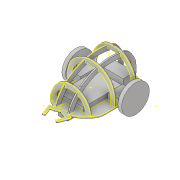
# Autodesk Inventor part: Chasis
Saved by Autodesk Inventor 2019 (Build 230136000, 136)
## iProperties
Created: 2019-02-16
Part Number: Chasis
Material: Generic
Document SubType Name: Modeling
Designer: carlg
Density: 1 g/cm^3
Appearance: Default
Author: carlg
Autodesk Inventor part; units mm, degrees
sketch "Sketch1" plane through (0, 0, 0) normal (0, 1, 0) x (-1, 0, 0)
  line L0 (0, 0) -> (-55.3, 0)
  line L1 (-55.3, 0) -> (-55.3, -83.15)
  line L2 (-55.3, -83.15) -> (0, -83.15)
  line L3 (0, -83.15) -> (0, 0)
  line L4 (-27.65, -83.15) -> (-27.65, 0) construction
  line L5 (-55.3, -83.15) -> (-55.3, 0)
  line L6 (-52.05, -89.15) -> (-3.25, -89.15)
  line L7 (-3.25, -89.15) -> (-3.25, -115.15)
  line L8 (-3.25, -115.15) -> (-52.05, -115.15)
  line L9 (-52.05, -115.15) -> (-52.05, -89.15)
  line L10 (-17.49, 2) -> (-37.81, 2)
  line L11 (-37.81, 2) -> (-37.81, 16.732)
  line L12 (-37.81, 16.732) -> (-17.49, 16.732)
  line L13 (-17.49, 16.732) -> (-17.49, 2)
  line L14 (-79.7, -83.15) -> (-79.7, -50.9)
  line L15 (-79.7, -68.4) -> (-84.2, -68.4)
  line L16 (-84.2, -68.4) -> (-84.2, -83.15)
  line L17 (-84.2, -83.15) -> (-79.7, -83.15)
  line L18 (-79.7, -65.65) -> (-79.7, -50.9)
  line L19 (-57.3, -83.15) -> (-79.7, -83.15)
  line L20 (-79.7, -50.9) -> (-57.3, -50.9)
  line L21 (-57.3, -83.15) -> (-57.3, -50.9)
  line L22 (-92.35, -75.775) -> (-92.35, -105.775)
  line L23 (-92.35, -105.775) -> (-84.2, -105.775)
  line L24 (-84.2, -105.775) -> (-84.2, -75.775)
  line L25 (-92.35, -75.775) -> (-92.35, -45.775)
  line L26 (-92.35, -45.775) -> (-84.2, -45.775)
  line L27 (-84.2, -45.775) -> (-84.2, -75.775)
  line L28 (2, -83.15) -> (2, -50.9)
  line L29 (2, -83.15) -> (24.4, -83.15)
  line L30 (24.4, -50.9) -> (2, -50.9)
  line L31 (24.4, -65.65) -> (24.4, -50.9)
  line L32 (24.4, -83.15) -> (24.4, -50.9)
  line L33 (24.4, -68.4) -> (28.9, -68.4)
  line L34 (28.9, -83.15) -> (24.4, -83.15)
  line L35 (28.9, -68.4) -> (28.9, -83.15)
  line L36 (37.05, -75.775) -> (37.05, -105.775)
  line L37 (37.05, -105.775) -> (28.9, -105.775)
  line L38 (28.9, -105.775) -> (28.9, -75.775)
  line L39 (37.05, -75.775) -> (37.05, -45.775)
  line L40 (37.05, -45.775) -> (28.9, -45.775)
  line L41 (28.9, -45.775) -> (28.9, -75.775)
  line L42 (-27.65, -119.15) -> (-27.65, -124.15)
  line L43 (2, -12.4357) -> (17.24, -12.4357)
  line L44 (17.24, -12.4357) -> (17.24, -40.9357)
  line L45 (17.24, -40.9357) -> (2, -40.9357)
  line L46 (2, -40.9357) -> (2, -12.4357)
  line L47 (0, 0) -> (2, 0)
  line L48 (-27.65, 16.732) -> (-27.65, 21.732)
  line L49 (-27.65, -124.15) -> (-27.65, 21.732)
  line L50 (24.4, -83.15) -> (2, -83.15)
  line L51 (2, -83.15) -> (2, -50.9)
  line L52 (2, -50.9) -> (24.4, -50.9)
  line L53 (24.4, -50.9) -> (24.4, -83.15)
  line L54 (-57.3, -83.15) -> (-79.7, -83.15)
  line L55 (-79.7, -83.15) -> (-79.7, -50.9)
  line L56 (-79.7, -50.9) -> (-57.3, -50.9)
  line L57 (-57.3, -50.9) -> (-57.3, -83.15)
  line L58 (28.9, -68.4) -> (24.4, -68.4)
  line L59 (24.4, -68.4) -> (24.4, -83.15)
  line L60 (24.4, -83.15) -> (28.9, -83.15)
  line L61 (28.9, -83.15) -> (28.9, -68.4)
  line L62 (-79.7, -68.4) -> (-84.2, -68.4)
  line L63 (-84.2, -68.4) -> (-84.2, -83.15)
  line L64 (-84.2, -83.15) -> (-79.7, -83.15)
  line L65 (-79.7, -83.15) -> (-79.7, -68.4)
  line L66 (-92.35, -75.775) -> (-84.2, -75.775)
  line L67 (-84.2, -75.775) -> (-84.2, -45.775)
  line L68 (-84.2, -45.775) -> (-92.35, -45.775)
  line L69 (-92.35, -45.775) -> (-92.35, -75.775)
  line L70 (37.05, -45.775) -> (28.9, -45.775)
  line L71 (28.9, -45.775) -> (28.9, -75.775)
  line L72 (28.9, -75.775) -> (37.05, -75.775)
  line L73 (37.05, -75.775) -> (37.05, -45.775)
  point P0 (-27.65, -93.15)
  point P1 (-27.65, -93.15)
  point P2 (-27.65, 2)
  point P3 (-27.65, 2)
  point P4 (-27.65, 2)
  point P5 (-27.65, 2)
  dimension "d100" = 32.315
  dimension "d0" = 83.15
  dimension "d1" = 55.3
  dimension "d7" = 26
  dimension "d8" = 48.8
  dimension "d9" = 10
  dimension "d12" = 6
  dimension "d14" = 30
  dimension "d15" = 30
  dimension "d16" = 8.15
  dimension "d17" = 20.32
  dimension "d18" = 14.732
  dimension "d19" = 2
  dimension "d21" = 2
  dimension "d22" = 2
  dimension "d24" = 5
  dimension "d25" = 15.24
  dimension "d26" = 28.5
  dimension "d27" = 2
  dimension "d28" = 5
  constraints: 148 end point, 22 parallel, 11 horizontal, 10 perpendicular, 5 midpoint, 3 vertical
  measures "d0" distance of L2.end L0.start
  measures "d1" distance of L0.start L0.end
  measures "d7" distance of L6.end L7.end
  measures "d8" distance of L6.start L6.end
  measures "d9" distance from line of L2 point (-27.65, -93.15)
  measures "d12" distance between parallel lines of L6 L2
  measures "d14" distance of L22.start L22.end
  measures "d15" distance of L25.start L25.end
  measures "d16" distance between parallel lines of L22 L24
  measures "d17" distance between parallel lines of L11 L13
  measures "d18" distance between parallel lines of L12 L10
  measures "d19" distance from line of L0 point (-27.65, 2)
  measures "d21" distance from line of L54.start L1
  measures "d22" distance of L2.end point (2, -83.15)
  measures "d24" distance of L42.start L42.end
  measures "d25" distance of L44.end L45.end
  measures "d26" distance of L43.end L44.end
  measures "d27" distance of L0.start L47.end
  measures "d28" distance of L48.start L48.end
sketch "Sketch2" plane through (0, 0, 0) normal (0, 1, 0) x (-1, 0, 0)
  line L0 (-79.7, -65.65) -> (-79.7, -50.9) projected
  line L1 (24.4, -65.65) -> (24.4, -50.9) projected
  line L2 (-79.7, -20.3869) -> (-79.7, -85.4945)
  line L3 (-27.65, 21.732) -> (-90.6639, 21.732)
  arc A0 (-27.65, 21.732) -> (-77.2994, -9.6974) centre (-27.6654, -33.1743) ccw
  line L4 (-27.65, -83.15) -> (-27.65, 0) construction
  line L5 (24.4, -20.3869) -> (24.4, -85.4945)
  arc A1 (21.9994, -9.6974) -> (-27.65, 21.732) centre (-27.6346, -33.1743) ccw
  arc A2 (-77.2994, -9.6974) -> (-79.7, -20.3869) centre (-54.7, -20.3869) ccw
  arc A3 (24.4, -20.3869) -> (21.9994, -9.6974) centre (-0.6, -20.3869) ccw
  line L6 (-27.65, -124.15) -> (-27.65, -129.15)
  line L7 (-27.65, -129.15) -> (30.0442, -129.15)
  arc A4 (-27.65, -129.15) -> (22.9704, -93.8274) centre (-26.988, -76.1656) ccw
  arc A5 (-78.2704, -93.8274) -> (-27.65, -129.15) centre (-28.312, -76.1656) ccw
  arc A6 (22.9704, -93.8274) -> (24.4, -85.4945) centre (-0.6, -85.4945) ccw
  arc A7 (-79.7, -85.4945) -> (-78.2704, -93.8274) centre (-54.7, -85.4945) ccw
  point P0 (0, 0)
  point P1 (-79.7, -83.15)
  point P2 (-37.81, 2)
  point P3 (-79.7, -15.65)
  point P4 (-27.65, -124.15)
  point P5 (24.4, -83.15)
  point P6 (24.4, -85.65)
  point P7 (24.4, -15.65)
  point P8 (-79.7, -89.0905)
  point P9 (24.4, -89.0905)
  dimension "d34" = 25
  dimension "d54" = 68.7036
  dimension "d55" = 5
  dimension "d56" = 68.7036
  dimension "d57" = 25
  constraints: 20 point on circle, 10 end point, 8 centre point, 8 tangent, 5 point on line, 4 symmetric about line, 2 horizontal, 2 vertical, 1 equal radius, 3 other
  measures "d34" radius of A2
  measures "d54" distance of L5.start point (24.4, -89.091)
  measures "d55" distance of L6.start L6.end
  measures "d56" distance of L2.start point (-79.7, -89.091)
  measures "d57" radius of A6
extrude "Extrusion1" add sketch "Sketch2" against normal blind 3.175
extrude "Extrusion2" add sketch "Sketch1" along normal blind 16.9 contours L6 L7 L8 L49 | L49 L8 L9 L6
extrude "Extrusion3" add sketch "Sketch1" along normal blind 10 contours L3 L2 L49 L0 | L49 L2 L1 L0
extrude "Extrusion4" add sketch "Sketch1" against normal blind 16.637 contours L10 L11 L12 L49 | L49 L12 L13 L10
extrude "Extrusion5" add sketch "Sketch1" along normal blind 1.75 contours L43 L44 L45 L46
extrude "Extrusion6" add sketch "Sketch1" along normal blind 12.8 contours L14 L20 L21 L19 | L28 L30 L31 L32 L29
extrude "Extrusion7" add sketch "Sketch1" along normal blind 12.8 contours L17 L16 L15 L14 | L32 L33 L35 L34
ref_plane "Work Plane1" through (0, 6.4, 0) normal (0, 1, 0) x (1, 0, 0)
sketch "Sketch3" plane through (0, 6.4, 0) normal (0, 1, 0) x (1, 0, 0)
  line L0 (-37.05, 75.775) -> (-37.05, 45.775) projected
  line L1 (-28.9, 75.775) -> (-37.05, 75.775) projected
  line L2 (-28.9, 45.775) -> (-28.9, 75.775) projected
  line L3 (-37.05, 45.775) -> (-28.9, 45.775) projected
  line L4 (92.35, 75.775) -> (84.2, 75.775) projected
  line L5 (92.35, 45.775) -> (84.2, 45.775) projected
  line L6 (84.2, 45.775) -> (84.2, 75.775) projected
  line L7 (92.35, 75.775) -> (92.35, 45.775) projected
  point P0 (0, 0)
revolve "Revolution1" add sketch "Sketch3" angle 360 about axis through (-28.9, 6.4, -75.775) along (-1, 0, 0) contours L1 L2 L3 L0
revolve "Revolution2" add sketch "Sketch3" angle 360 about axis through (92.35, 6.4, -75.775) along (-1, 0, 0) contours L7 L5 L6 L4
sketch "Sketch5" plane through (0, 0, 0) normal (0, 1, 0) x (1, 0, 0)
  line L0 (37.81, -16.732) -> (37.81, -2) projected
  line L1 (17.49, -2) -> (17.49, -16.732) projected
  line L2 (37.81, -9.366) -> (39.81, -9.366)
  arc A0 (-21.9994, 9.6974) -> (27.65, -21.732) centre (27.6346, 33.1743) ccw projected
  arc A1 (-21.9994, 9.6974) -> (27.65, -21.732) centre (27.6346, 33.1743) ccw projected
  line L3 (12.315, -18.525) -> (12.315, -9)
  line L4 (12.315, -9) -> (15.49, -9)
  line L5 (15.49, -9) -> (15.49, -18.525)
  line L6 (15.49, -18.525) -> (12.315, -18.525)
  line L7 (12.315, -18.525) -> (12.315, -9)
  arc A2 (27.65, 129.15) -> (-22.9704, 93.8274) centre (26.988, 76.1656) ccw projected
  line L8 (27.65, -21.732) -> (27.65, 129.15) construction
  line L9 (42.985, -17.0839) -> (42.985, -14.4607)
  line L10 (42.985, -18.525) -> (42.985, -9)
  line L11 (42.985, -9) -> (39.81, -9)
  line L12 (39.81, -9) -> (39.81, -18.525)
  line L13 (39.81, -18.525) -> (42.985, -18.525)
  line L14 (42.985, -18.525) -> (42.985, -9)
  line L15 (27.65, 53.709) -> (108.4931, 53.709)
  line L16 (0, 0) -> (55.3, 0) projected
  line L17 (12.315, 125.943) -> (12.315, 116.418)
  line L18 (12.315, 116.418) -> (15.49, 116.418)
  line L19 (15.49, 116.418) -> (15.49, 125.943)
  line L20 (15.49, 125.943) -> (12.315, 125.943)
  line L21 (42.985, 125.943) -> (42.985, 116.418)
  line L22 (42.985, 116.418) -> (39.81, 116.418)
  line L23 (39.81, 116.418) -> (39.81, 125.943)
  line L24 (39.81, 125.943) -> (42.985, 125.943)
  line L25 (41.3975, -9) -> (41.3975, -7.3761)
  point P0 (12.315, -19.5515)
  point P1 (42.985, -19.5515)
  dimension "d58" = 2
  dimension "d64" = 9
  dimension "d65" = 3.175
  dimension "d66" = 2
  dimension "d67" = 9.525
  dimension "d71" = 13.7475
  constraints: 46 end point, 13 symmetric about line, 3 horizontal, 3 midpoint, 3 vertical, 2 parallel, 1 perpendicular, 1 point on circle
  measures "d58" distance of L2.start L2.end
  measures "d64" distance between parallel lines of L4 L16
  measures "d65" distance between parallel lines of L5 L3
  measures "d66" distance between parallel lines of L1 L5
  measures "d67" distance between parallel lines of L4 L6
  measures "d71" distance between parallel lines of L8 L25
ref_plane "Work Plane3" through (27.65, -3.175, -20.3869) normal (1, 0, 0) x (0, 0, -1)
sketch "Sketch6" plane through (27.65, -3.175, -20.3869) normal (1, 0, 0) x (0, 0, -1)
  line L0 (-29.3869, 3.175) -> (-38.9119, 3.175) projected
  line L1 (96.0311, 3.175) -> (105.5561, 3.175) projected
  arc A0 (-6.8223, 33.7853) -> (-29.3869, 3.175) centre (34.2192, -20.0908) ccw
  arc A1 (96.0311, 3.175) -> (96.0508, 28.0481) centre (-63.3442, 15.738) ccw
  arc A2 (95.7943, 29.288) -> (84.7823, 48.1242) centre (43.3553, 11.2684) ccw
  arc A3 (79.8048, 51.1614) -> (-6.8223, 33.7853) centre (54.4776, -47.1959) ccw
  arc A4 (84.7823, 48.1242) -> (79.8048, 51.1614) centre (77.3111, 41.4773) ccw
  arc A5 (96.0508, 28.0481) -> (95.7943, 29.288) centre (91.0656, 27.6631) ccw
  arc A6 (-12.5825, 41.3712) -> (-35.7289, 12.7) centre (34.2192, -20.0908) ccw
  arc A7 (82.18, 60.3855) -> (-12.5825, 41.3712) centre (54.4776, -47.1959) ccw
  arc A8 (91.8987, 54.4553) -> (82.18, 60.3855) centre (77.3111, 41.4773) ccw
  arc A9 (104.8022, 32.3835) -> (91.8987, 54.4553) centre (43.3553, 11.2684) ccw
  arc A10 (105.5475, 28.7816) -> (104.8022, 32.3835) centre (91.0656, 27.6631) ccw
  arc A11 (106.0232, 12.7) -> (105.5475, 28.7816) centre (-63.3442, 15.738) ccw
  arc A12 (-35.7289, 12.7) -> (-38.9119, 3.175) centre (0.5043, -4.7026) ccw
  arc A13 (105.5561, 3.175) -> (106.0232, 12.7) centre (-43.7923, 15.2735) ccw
  point P0 (-20.3869, 3.175)
  dimension "d68" = 10
  dimension "d69" = 5
  dimension "d70" = 9.525
  constraints: 28 point on circle, 14 centre point, 4 tangent, 5 other
  measures "d68" radius of A4
  measures "d69" radius of A5
  measures "d70" radial gap between concentric circles of A3 A7
ref_plane "Work Plane4" through (41.398, -3.175, -20.3869) normal (1, 0, 0) x (0, 0, -1)
sketch "Sketch7" plane through (41.398, -3.175, -20.3869) normal (1, 0, 0) x (0, 0, -1)
  arc A0 (82.18, 60.3855) -> (-12.5825, 41.3712) centre (54.4776, -47.1959) ccw projected
  arc A1 (-12.5825, 41.3712) -> (-35.7289, 12.7) centre (34.2192, -20.0908) ccw projected
  arc A2 (-35.7289, 12.7) -> (-38.9119, 3.175) centre (0.5043, -4.7026) ccw projected
  arc A3 (-6.8223, 33.7853) -> (-29.3869, 3.175) centre (34.2192, -20.0908) ccw projected
  arc A4 (79.8048, 51.1614) -> (-6.8223, 33.7853) centre (54.4776, -47.1959) ccw projected
  arc A5 (84.7823, 48.1242) -> (79.8048, 51.1614) centre (77.3111, 41.4773) ccw projected
  arc A6 (95.7943, 29.288) -> (84.7823, 48.1242) centre (43.3553, 11.2684) ccw projected
  arc A7 (96.0311, 3.175) -> (96.0508, 28.0481) centre (-63.3442, 15.738) ccw projected
  arc A8 (106.0232, 12.7) -> (105.5475, 28.7816) centre (-63.3442, 15.738) ccw projected
  arc A9 (105.5561, 3.175) -> (106.0232, 12.7) centre (-43.7923, 15.2735) ccw projected
  arc A10 (104.8022, 32.3835) -> (91.8987, 54.4553) centre (43.3553, 11.2684) ccw projected
  arc A11 (105.5475, 28.7816) -> (104.8022, 32.3835) centre (91.0656, 27.6631) ccw projected
  arc A12 (91.8987, 54.4553) -> (82.18, 60.3855) centre (77.3111, 41.4773) ccw projected
  line L0 (-38.9119, 3.175) -> (-29.3869, 3.175)
  line L1 (96.0311, 3.175) -> (105.5561, 3.175)
  line L2 (-38.9119, 3.175) -> (-29.3869, 3.175)
  line L3 (96.0311, 3.175) -> (105.5561, 3.175)
  arc A13 (96.0508, 28.0481) -> (95.7943, 29.288) centre (91.0656, 27.6631) ccw projected
  point P0 (-20.3869, 3.175)
  point P1 (108.7631, 3.175)
  constraints: 8 end point, 2 collinear
extrude "Extrusion8" add sketch "Sketch7" along normal mid plane 3.048
mirror "Mirror1" about plane through (27.65, -3.175, -20.3869) normal (1, 0, 0) of "Extrusion8"
sketch "Sketch8" plane through (0, 0, 0) normal (0, 1, 0) x (1, 0, 0)
  line L0 (-21.275, 92.15) -> (-11.75, 92.15)
  line L1 (-11.75, 92.15) -> (-11.75, 95.325)
  line L2 (-11.75, 95.325) -> (-21.275, 95.325)
  line L3 (-21.275, 95.325) -> (-21.275, 92.15)
  line L4 (-2, 83.15) -> (-28.9, 83.15) projected
  line L5 (3.25, 115.15) -> (3.25, 89.15) projected
  line L6 (-23.275, 46.9) -> (-13.75, 46.9)
  line L7 (-13.75, 46.9) -> (-13.75, 43.725)
  line L8 (-13.75, 43.725) -> (-23.275, 43.725)
  line L9 (-23.275, 43.725) -> (-23.275, 46.9)
  line L10 (-24.4, 50.9) -> (-2, 50.9) projected
  line L11 (-14.525, 0.2607) -> (-5, 0.2607)
  line L12 (-5, 0.2607) -> (-5, 3.4357)
  line L13 (-5, 3.4357) -> (-14.525, 3.4357)
  line L14 (-14.525, 3.4357) -> (-14.525, 0.2607)
  line L15 (0, 83.15) -> (0, 0) projected
  line L16 (-17.24, 12.4357) -> (-2, 12.4357) projected
  line L17 (27.65, -21.732) -> (27.65, 129.15) construction
  line L18 (76.575, 92.15) -> (67.05, 92.15)
  line L19 (67.05, 92.15) -> (67.05, 95.325)
  line L20 (67.05, 95.325) -> (76.575, 95.325)
  line L21 (76.575, 95.325) -> (76.575, 92.15)
  line L22 (57.3, 83.15) -> (84.2, 83.15)
  line L23 (78.575, 46.9) -> (69.05, 46.9)
  line L24 (69.05, 46.9) -> (69.05, 43.725)
  line L25 (69.05, 43.725) -> (78.575, 43.725)
  line L26 (78.575, 43.725) -> (78.575, 46.9)
  line L27 (79.7, 50.9) -> (57.3, 50.9)
  line L28 (69.825, 0.2607) -> (60.3, 0.2607)
  line L29 (60.3, 0.2607) -> (60.3, 3.4357)
  line L30 (60.3, 3.4357) -> (69.825, 3.4357)
  line L31 (69.825, 3.4357) -> (69.825, 0.2607)
  line L32 (72.54, 12.4357) -> (57.3, 12.4357)
  line L33 (-5, 1.8482) -> (-2.9235, 1.8482)
  line L34 (0, 0) -> (55.3, 0) projected
  line L35 (-13.75, 45.3125) -> (-11.75, 45.3125)
  line L36 (-2, 40.9357) -> (-17.24, 40.9357) projected
  dimension "d75" = 3.175
  dimension "d76" = 9
  dimension "d77" = 9.525
  dimension "d78" = 15
  dimension "d79" = 9.525
  dimension "d80" = 3.175
  dimension "d81" = 4
  dimension "d82" = 9.525
  dimension "d83" = 3.175
  dimension "d84" = 5
  dimension "d85" = 9
  dimension "d86" = 13.75
  dimension "d87" = 1.8482
  dimension "d89" = 4.3768
  constraints: 58 end point, 18 symmetric about line, 6 parallel, 5 horizontal, 3 perpendicular, 2 midpoint
  measures "d75" distance of L2.end L0.start
  measures "d76" distance between parallel lines of L0 L4
  measures "d77" distance of L1.end L2.end
  measures "d78" distance between parallel lines of L5 L1
  measures "d79" distance between parallel lines of L7 L9
  measures "d80" distance between parallel lines of L6 L8
  measures "d81" distance between parallel lines of L10 L6
  measures "d82" distance of L12.end L13.end
  measures "d83" distance between parallel lines of L13 L11
  measures "d84" distance between parallel lines of L15 L12
  measures "d85" distance between parallel lines of L16 L13
  measures "d86" distance between parallel lines of L15 L7
  measures "d87" distance between parallel lines of L33 L34
  measures "d89" distance between parallel lines of L36 L35
ref_plane "Work Plane5" through (0, 0, -1.848) normal (0, 0, 1) x (1, 0, 0)
ref_plane "Work Plane6" through (-2, 0, -45.3127) normal (0, 0, -1) x (-1, 0, 0)
ref_plane "Work Plane7" through (-2, 0, -93.7375) normal (0, 0, -1) x (-1, 0, 0)
sketch "Sketch10" plane through (-2, 0, -45.3127) normal (0, 0, -1) x (-1, 0, 0)
  line L0 (-80.575, 0) -> (-71.05, 0) projected
  line L1 (21.275, 0) -> (11.75, 0) projected
  point P0 (-2, 0)
sketch "Sketch11" plane through (-2, 0, -93.7375) normal (0, 0, -1) x (-1, 0, 0)
  line L0 (9.75, 0) -> (19.275, 0) projected
  line L1 (-69.05, 0) -> (-78.575, 0) projected
  point P0 (-2, 0)
ref_plane "Work Plane8" through (0, 0, -1.848) normal (0, 0, 1) x (1, 0, 0)
sketch "Sketch13" plane through (0, 0, -1.848) normal (0, 0, 1) x (1, 0, 0)
  line L0 (60.3, 0) -> (69.825, 0) projected
  line L1 (-5, 0) -> (-14.525, 0) projected
  line L2 (15.426, 26.113) -> (12.378, 26.113) projected
  line L3 (42.922, 30.6103) -> (42.922, 30.6103) projected
  line L4 (42.922, 51.195) -> (42.922, 30.6103) projected
  arc A0 (29.345, 28.3859) -> (-5, 0) centre (27.0848, -3.85) ccw
  arc A1 (60.3, 0) -> (29.345, 28.3859) centre (28.2224, -3.9096) ccw
  line L5 (-14.525, 0) -> (-5, 0)
  line L6 (-2, 1.75) -> (-17.24, 1.75) projected
  line L7 (60.3, 0) -> (69.825, 0)
  line L8 (57.3, 0) -> (79.7, 0) projected
  arc A2 (67.8468, 9.525) -> (29.6759, 37.9051) centre (28.2224, -3.9096) ccw
  line L9 (27.65, 0) -> (27.65, -3.175) projected
  line L10 (27.65, 0) -> (27.65, 24.5505)
  arc A3 (25.6241, 37.9051) -> (-12.5468, 9.525) centre (27.0776, -3.9096) ccw
  arc A4 (29.6759, 37.9051) -> (25.6241, 37.9051) centre (27.65, 13.4592) ccw
  arc A5 (-12.5468, 9.525) -> (-14.525, 0) centre (24.7018, -3.1788) ccw
  arc A6 (69.825, 0) -> (67.8468, 9.525) centre (30.5982, -3.1788) ccw
  point P0 (0, 0)
  point P1 (42.922, 47.9864)
  point P2 (69.8793, 0)
  dimension "d100" = 32.315
  dimension "d116" = 9.525
  constraints: 15 point on circle, 7 centre point, 6 end point, 4 symmetric about line, 1 collinear, 1 parallel, 1 point on line, 1 vertical, 3 other
  measures "d100" radius of A0
  measures "d116" radial gap between concentric circles of A1 A2
extrude "Extrusion10" add sketch "Sketch13" along normal mid plane 3.048
ref_plane "Work Plane9" through (-2, 0, -45.3127) normal (0, 0, 1) x (1, 0, 0)
sketch "Sketch16" plane through (-2, 0, -45.3127) normal (0, 0, 1) x (1, 0, 0)
  line L0 (-21.275, 0) -> (-11.75, 0) projected
  line L1 (80.575, 0) -> (71.05, 0) projected
  line L2 (17.426, 30.6103) -> (17.426, 51.195) projected
  line L3 (41.874, 30.6103) -> (41.874, 51.195) projected
  line L4 (44.922, 51.195) -> (41.874, 51.195) projected
  arc A0 (29.7378, 52.9646) -> (-11.75, 0) centre (28.7906, 10.9752) ccw
  arc A1 (-15.1613, 37.8649) -> (-21.275, 0) centre (49.5076, 7.9974) ccw
  line L5 (-21.275, 0) -> (-11.75, 0)
  line L6 (80.575, 0) -> (71.05, 0)
  arc A2 (71.05, 0) -> (29.5626, 52.9631) centre (30.5089, 10.9737) ccw
  arc A3 (74.4622, 37.8642) -> (28.0459, 62.4413) centre (30.5089, 10.9737) ccw
  arc A4 (80.575, 0) -> (74.4622, 37.8642) centre (9.7925, 7.9983) ccw
  line L7 (71.05, 0) -> (80.575, 0)
  line L8 (-11.75, 0) -> (-21.275, 0)
  line L9 (-21.275, 0) -> (-11.75, 0)
  line L10 (71.05, 0) -> (80.575, 0)
  arc A5 (29.5626, 52.9631) -> (-11.75, 0) centre (28.7868, 10.9742) ccw
  arc A6 (71.05, 0) -> (29.5626, 52.9631) centre (30.5089, 10.9737) ccw
  arc A7 (80.575, 0) -> (74.4622, 37.8642) centre (9.7925, 7.9983) ccw
  arc A8 (74.4622, 37.8642) -> (28.0459, 62.4413) centre (30.5089, 10.9737) ccw
  arc A9 (-15.1613, 37.8649) -> (-21.275, 0) centre (49.5076, 7.9974) ccw
  line L11 (29.3469, 65.1955) -> (29.3469, 72.5877)
  arc A10 (28.0459, 62.4413) -> (-15.1613, 37.8649) centre (30.6726, 7.5545) ccw
  point P0 (2, 0)
  point P1 (17.426, 47.9864)
  point P2 (41.874, 47.9864)
  dimension "d119" = 42
  constraints: 23 point on circle, 14 end point, 11 centre point, 3 collinear, 3 concentric, 3 tangent, 1 horizontal, 1 vertical
  measures "d119" radius of A0
extrude "Extrusion14" add sketch "Sketch16" along normal mid plane 3.048 contours A1 A10 A3 A4 L1 A2 A0 L0
sketch "Sketch17" plane through (-2, 0, -93.7375) normal (0, 0, -1) x (-1, 0, 0)
  line L0 (9.75, 0) -> (19.275, 0) projected
  line L1 (-69.05, 0) -> (-78.575, 0) projected
  line L2 (19.275, 0) -> (9.75, 0)
  line L3 (-17.426, 57.1262) -> (-17.426, 60.72) projected
  line L4 (-17.426, 58.9231) -> (-41.874, 58.9231)
  line L5 (-41.874, 57.1262) -> (-41.874, 60.72) projected
  line L6 (-29.65, 58.9231) -> (-29.65, 52.1907)
  arc A0 (-14.5459, 53.0039) -> (-29.65, 55.5569) centre (-28.9804, 13.5622) ccw
  line L7 (-14.378, 57.2105) -> (-14.378, 51.2803) projected
  arc A1 (9.75, 0) -> (-12.959, 52.1799) centre (-43.8415, 7.7082) ccw
  arc A2 (-12.959, 52.1799) -> (-14.5459, 53.0039) centre (-16.9517, 46.4303) ccw
  arc A3 (-29.65, 55.5569) -> (-44.7541, 53.0039) centre (-30.3196, 13.5622) ccw
  arc A4 (-46.341, 52.1799) -> (-69.05, 0) centre (-15.4585, 7.7082) ccw
  arc A5 (-44.7541, 53.0039) -> (-46.341, 52.1799) centre (-42.3483, 46.4303) ccw
  arc A6 (-51.774, 60.0035) -> (-75.1717, 29.7979) centre (-15.4585, 7.7082) ccw
  arc A7 (-48.0276, 61.9487) -> (-51.774, 60.0035) centre (-42.3483, 46.4303) ccw
  arc A8 (-29.65, 65.0829) -> (-48.0276, 61.9487) centre (-30.3196, 13.5622) ccw
  arc A9 (-11.2724, 61.9487) -> (-29.65, 65.0829) centre (-28.9804, 13.5622) ccw
  arc A10 (-7.526, 60.0035) -> (-11.2724, 61.9487) centre (-16.9517, 46.4303) ccw
  arc A11 (15.8717, 29.7979) -> (-7.526, 60.0035) centre (-43.8415, 7.7082) ccw
  arc A12 (19.275, 0) -> (16.153, 28.8269) centre (-123.2548, -0.8536) ccw
  arc A13 (-75.453, 28.8269) -> (-78.575, 0) centre (63.9548, -0.8536) ccw
  arc A14 (16.153, 28.8269) -> (15.8717, 29.7979) centre (9.3065, 27.3692) ccw
  arc A15 (-75.1717, 29.7979) -> (-75.453, 28.8269) centre (-68.6065, 27.3692) ccw
  point P0 (-2, 0)
  point P1 (-17.426, 57.2105)
  point P2 (-41.874, 57.2105)
  dimension "d124" = 42
  dimension "d125" = 7
  dimension "d126" = 9.525
  dimension "d127" = 7
  constraints: 32 point on circle, 16 centre point, 6 end point, 6 symmetric about line, 6 tangent, 4 midpoint, 1 collinear, 1 equal radius, 1 vertical, 7 other
  measures "d124" radius of A0
  measures "d125" radius of A2
  measures "d126" radial gap between concentric circles of A3 A8
  measures "d127" radius of A14
extrude "Extrusion15" add sketch "Sketch17" along normal mid plane 3.048
sketch "Sketch18" plane through (0, -3.175, 0) normal (0, -1, 0) x (1, 0, 0)
  line L0 (17.49, 2) -> (17.49, 16.732) projected
  line L1 (17.49, 16.732) -> (37.81, 16.732) projected
  line L2 (37.81, 16.732) -> (37.81, 2) projected
  line L3 (37.81, 2) -> (17.49, 2) projected
  arc A0 (77.2994, -9.6974) -> (27.65, 21.732) centre (27.6654, -33.1743) ccw projected
  arc A1 (27.65, 21.732) -> (-21.9994, -9.6974) centre (27.6346, -33.1743) ccw projected
  arc A2 (-21.9994, -9.6974) -> (-24.4, -20.3869) centre (0.6, -20.3869) ccw projected
  line L4 (-24.4, -20.3869) -> (-24.4, -85.4945) projected
  arc A3 (-24.4, -85.4945) -> (-22.9704, -93.8274) centre (0.6, -85.4945) ccw projected
  arc A4 (-22.9704, -93.8274) -> (27.65, -129.15) centre (26.988, -76.1656) ccw projected
  arc A5 (27.65, -129.15) -> (78.2704, -93.8274) centre (28.312, -76.1656) ccw projected
  arc A6 (78.2704, -93.8274) -> (79.7, -85.4945) centre (54.7, -85.4945) ccw projected
  line L5 (79.7, -85.4945) -> (79.7, -20.3869) projected
  arc A7 (79.7, -20.3869) -> (77.2994, -9.6974) centre (54.7, -20.3869) ccw projected
  arc A8 (27.65, 21.732) -> (-21.9994, -9.6974) centre (27.6346, -33.1743) ccw projected
  line L6 (27.65, 21.732) -> (27.65, 17.7013)
  arc A9 (77.2994, -9.6974) -> (27.65, 21.732) centre (27.6654, -33.1743) ccw projected
  line L7 (27.2302, 21.9261) -> (18.5737, 25.9296)
  line L8 (16.4748, 21.3915) -> (22.65, 18.5356)
  line L9 (22.65, 18.5356) -> (22.65, 17.7013)
  line L10 (22.65, 18.5356) -> (4.1968, 22.1506)
  line L11 (3.4573, 23.495) -> (11.7364, 44.743)
  line L12 (13.0312, 45.3117) -> (15.8265, 44.2226)
  line L13 (16.3952, 42.9278) -> (10.8305, 28.6461)
  line L14 (11.57, 27.3017) -> (18.5737, 25.9296)
  line L15 (28.0698, 21.9261) -> (36.7263, 25.9296)
  line L16 (38.8252, 21.3915) -> (32.65, 18.5356)
  line L17 (32.65, 18.5356) -> (32.65, 17.7013)
  line L18 (32.65, 18.5356) -> (51.1032, 22.1506)
  line L19 (51.8427, 23.495) -> (43.5636, 44.743)
  line L20 (42.2688, 45.3117) -> (39.4735, 44.2226)
  line L21 (38.9048, 42.9278) -> (44.4695, 28.6461)
  line L22 (43.73, 27.3017) -> (36.7263, 25.9296)
  line L23 (22.65, 17.7013) -> (32.65, 17.7013)
  arc A10 (13.0312, 45.3117) -> (11.7364, 44.743) centre (12.6681, 44.38) ccw
  arc A11 (16.3952, 42.9278) -> (15.8265, 44.2226) centre (15.4634, 43.2908) ccw
  arc A12 (10.8305, 28.6461) -> (11.57, 27.3017) centre (11.7623, 28.283) ccw
  arc A13 (3.4573, 23.495) -> (4.1968, 22.1506) centre (4.3891, 23.132) ccw
  arc A14 (27.2302, 21.9261) -> (28.0698, 21.9261) centre (27.65, 22.8338) ccw
  arc A15 (43.73, 27.3017) -> (44.4695, 28.6461) centre (43.5377, 28.283) ccw
  arc A16 (39.4735, 44.2226) -> (38.9048, 42.9278) centre (39.8366, 43.2908) ccw
  arc A17 (43.5636, 44.743) -> (42.2688, 45.3117) centre (42.6319, 44.38) ccw
  arc A18 (51.1032, 22.1506) -> (51.8427, 23.495) centre (50.9109, 23.132) ccw
  point P0 (0, 0)
  point P1 (3.0231, 22.3806)
  point P2 (12.0994, 45.6748)
  point P3 (16.7583, 43.8595)
  point P4 (10.3963, 27.5316)
  point P5 (52.2769, 22.3806)
  point P6 (43.2006, 45.6748)
  point P7 (38.5417, 43.8595)
  point P8 (44.9037, 27.5316)
  dimension "d130" = 10
  dimension "d131" = 5
  dimension "d132" = 20
  dimension "d133" = 25
  dimension "d134" = 5
  dimension "d135" = 1
  constraints: 36 end point, 18 point on circle, 18 point on line, 18 tangent, 9 centre point, 8 equal radius, 8 symmetric about line, 2 parallel, 2 perpendicular, 1 vertical, 1 other
  measures "d130" distance of L6.start L7.end
  measures "d131" distance between parallel lines of L7 L8
  measures "d132" distance of L8.end point (3.023, 22.381)
  measures "d133" distance of point (3.023, 22.381) point (12.099, 45.675)
  measures "d134" distance of point (12.099, 45.675) point (16.758, 43.86)
  measures "d135" radius of A10
extrude "Extrusion16" add sketch "Sketch18" against normal blind 3.175 contours L18 L16 A0 | A0 A1 L10 A13 L11 A10 L12 A11 L13 A12 L14 L7 A14 L15 L22 A15 L21 A16 L20 A17 L19 A18 L18 | L16 L17 L23 L6 A0 | L6 L23 L9 L8 A1 | L8 L10 A1
sketch "Sketch20" plane through (0, 0, 0) normal (0, 1, 0) x (1, 0, 0)
  arc A0 (40.8128, -20.1347) -> (77.2994, 9.6974) centre (27.6654, 33.1743) ccw projected
  arc A1 (77.2994, 9.6974) -> (79.7, 20.3869) centre (54.7, 20.3869) ccw projected
  line L0 (79.7, 20.3869) -> (79.7, 50.9) projected
  line L1 (79.7, 50.9) -> (57.3, 50.9) projected
  line L2 (57.3, 50.9) -> (57.3, 83.15) projected
  line L3 (57.3, 83.15) -> (79.7, 83.15) projected
  line L4 (79.7, 83.15) -> (79.7, 85.4945) projected
  arc A2 (79.7, 85.4945) -> (78.2704, 93.8274) centre (54.7, 85.4945) ccw projected
  arc A3 (78.2704, 93.8274) -> (27.65, 129.15) centre (28.312, 76.1656) ccw projected
  arc A4 (27.65, 129.15) -> (-22.9704, 93.8274) centre (26.988, 76.1656) ccw projected
  arc A5 (-22.9704, 93.8274) -> (-24.4, 85.4945) centre (0.6, 85.4945) ccw projected
  line L5 (-24.4, 85.4945) -> (-24.4, 83.15) projected
  line L6 (-24.4, 83.15) -> (-2, 83.15) projected
  line L7 (-2, 83.15) -> (-2, 50.9) projected
  line L8 (-2, 50.9) -> (-24.4, 50.9) projected
  line L9 (-24.4, 50.9) -> (-24.4, 20.3869) projected
  arc A6 (-24.4, 20.3869) -> (-21.9994, 9.6974) centre (0.6, 20.3869) ccw projected
  arc A7 (-21.9994, 9.6974) -> (14.4872, -20.1347) centre (27.6346, 33.1743) ccw projected
  line L10 (14.4872, -20.1347) -> (4.1968, -22.1506) projected
  arc A8 (4.1968, -22.1506) -> (3.4573, -23.495) centre (4.3891, -23.132) ccw projected
  line L11 (3.4573, -23.495) -> (11.7364, -44.743) projected
  arc A9 (11.7364, -44.743) -> (13.0312, -45.3117) centre (12.6681, -44.38) ccw projected
  line L12 (13.0312, -45.3117) -> (15.8265, -44.2226) projected
  arc A10 (15.8265, -44.2226) -> (16.3952, -42.9278) centre (15.4634, -43.2908) ccw projected
  line L13 (16.3952, -42.9278) -> (10.8305, -28.6461) projected
  arc A11 (11.57, -27.3017) -> (10.8305, -28.6461) centre (11.7623, -28.283) ccw projected
  line L14 (11.57, -27.3017) -> (18.5737, -25.9296) projected
  line L15 (18.5737, -25.9296) -> (27.2302, -21.9261) projected
  arc A12 (28.0698, -21.9261) -> (27.2302, -21.9261) centre (27.65, -22.8338) ccw projected
  line L16 (28.0698, -21.9261) -> (36.7263, -25.9296) projected
  line L17 (36.7263, -25.9296) -> (43.73, -27.3017) projected
  arc A13 (44.4695, -28.6461) -> (43.73, -27.3017) centre (43.5377, -28.283) ccw projected
  line L18 (44.4695, -28.6461) -> (38.9048, -42.9278) projected
  arc A14 (38.9048, -42.9278) -> (39.4735, -44.2226) centre (39.8366, -43.2908) ccw projected
  line L19 (39.4735, -44.2226) -> (42.2688, -45.3117) projected
  arc A15 (42.2688, -45.3117) -> (43.5636, -44.743) centre (42.6319, -44.38) ccw projected
  line L20 (43.5636, -44.743) -> (51.8427, -23.495) projected
  arc A16 (51.8427, -23.495) -> (51.1032, -22.1506) centre (50.9109, -23.132) ccw projected
  line L21 (51.1032, -22.1506) -> (40.8128, -20.1347) projected
  line L22 (76.575, 92.2135) -> (67.05, 92.2135) projected
  line L23 (67.05, 92.2135) -> (67.05, 95.2615) projected
  line L24 (67.05, 95.2615) -> (76.575, 95.2615) projected
  line L25 (76.575, 95.2615) -> (76.575, 92.2135) projected
  line L26 (-11.75, 92.2135) -> (-21.275, 92.2135) projected
  line L27 (-21.275, 92.2135) -> (-21.275, 95.2615) projected
  line L28 (-21.275, 95.2615) -> (-11.75, 95.2615) projected
  line L29 (-11.75, 95.2615) -> (-11.75, 92.2135) projected
  line L30 (-23.275, 46.8367) -> (-13.75, 46.8367) projected
  line L31 (-13.75, 46.8367) -> (-13.75, 43.7887) projected
  line L32 (-13.75, 43.7887) -> (-23.275, 43.7887) projected
  line L33 (-23.275, 43.7887) -> (-23.275, 46.8367) projected
  line L34 (69.05, 46.8367) -> (78.575, 46.8367) projected
  line L35 (78.575, 46.8367) -> (78.575, 43.7887) projected
  line L36 (78.575, 43.7887) -> (69.05, 43.7887) projected
  line L37 (69.05, 43.7887) -> (69.05, 46.8367) projected
  line L38 (-14.525, 3.372) -> (-5, 3.372) projected
  line L39 (-5, 3.372) -> (-5, 0.324) projected
  line L40 (-5, 0.324) -> (-14.525, 0.324) projected
  line L41 (-14.525, 0.324) -> (-14.525, 3.372) projected
  line L42 (60.3, 3.372) -> (69.825, 3.372) projected
  line L43 (69.825, 3.372) -> (69.825, 0.324) projected
  line L44 (69.825, 0.324) -> (60.3, 0.324) projected
  line L45 (60.3, 0.324) -> (60.3, 3.372) projected
  line L46 (15.426, 125.943) -> (15.426, 116.418) projected
  line L47 (15.426, 116.418) -> (12.378, 116.418) projected
  line L48 (12.378, 116.418) -> (12.378, 125.943) projected
  line L49 (12.378, 125.943) -> (15.426, 125.943) projected
  line L50 (15.426, -9) -> (15.426, -18.525) projected
  line L51 (15.426, -18.525) -> (12.378, -18.525) projected
  line L52 (12.378, -18.525) -> (12.378, -9) projected
  line L53 (12.378, -9) -> (15.426, -9) projected
  line L54 (39.874, -18.525) -> (39.874, -9) projected
  line L55 (39.874, -9) -> (42.922, -9) projected
  line L56 (42.922, -9) -> (42.922, -18.525) projected
  line L57 (42.922, -18.525) -> (39.874, -18.525) projected
  line L58 (39.874, 116.418) -> (39.874, 125.943) projected
  line L59 (39.874, 125.943) -> (42.922, 125.943) projected
  line L60 (42.922, 125.943) -> (42.922, 116.418) projected
  line L61 (42.922, 116.418) -> (39.874, 116.418) projected
  line L62 (3.25, 89.15) -> (3.25, 115.15) projected
  line L63 (3.25, 115.15) -> (52.05, 115.15) projected
  line L64 (52.05, 115.15) -> (52.05, 89.15) projected
  line L65 (52.05, 89.15) -> (3.25, 89.15) projected
  line L66 (0, 0) -> (0, 83.15) projected
  line L67 (0, 83.15) -> (55.3, 83.15) projected
  line L68 (55.3, 83.15) -> (55.3, 0) projected
  line L69 (55.3, 0) -> (0, 0) projected
  line L70 (-17.24, 12.4357) -> (-17.24, 40.9357) projected
  line L71 (-17.24, 40.9357) -> (-2, 40.9357) projected
  line L72 (-2, 40.9357) -> (-2, 12.4357) projected
  line L73 (-2, 12.4357) -> (-17.24, 12.4357) projected
  line L74 (17.49, -2) -> (37.81, -2) projected
  line L75 (37.81, -2) -> (37.81, -16.732) projected
  line L76 (37.81, -16.732) -> (17.49, -16.732) projected
  line L77 (17.49, -16.732) -> (17.49, -2) projected
  line L78 (79.7, 85.4945) -> (79.7, 20.3869) projected
  line L79 (-24.4, 20.3869) -> (-24.4, 85.4945) projected
sketch "Sketch21" plane through (12.378, 0, -125.943) normal (-1, 0, 0) x (0, 0, 1)
  line L0 (30.6815, 52.94) -> (30.6815, 58.8314) projected
  arc A0 (30.6815, 58.8314) -> (23.3761, 57.2105) centre (51.0785, -50.3709) ccw projected
  arc A1 (23.3761, 57.2105) -> (13.6574, 51.2803) centre (28.245, 38.3023) ccw projected
  arc A2 (13.6574, 51.2803) -> (0.7538, 29.2085) centre (62.2007, 8.0934) ccw projected
  arc A3 (0.7538, 29.2085) -> (0.0085, 25.6066) centre (14.4904, 24.4881) ccw projected
  arc A4 (0.0085, 25.6066) -> (-0.4671, 9.525) centre (168.9002, 12.563) ccw projected
  arc A5 (-0.4671, 9.525) -> (0, 0) centre (149.3484, 12.0985) ccw projected
  line L1 (9.525, 0) -> (0, 0) projected
  arc A6 (9.5053, 24.8731) -> (9.525, 0) centre (168.9002, 12.563) ccw projected
  arc A7 (9.7618, 26.113) -> (9.5053, 24.8731) centre (14.4904, 24.4881) ccw projected
  arc A8 (20.7737, 44.9492) -> (9.7618, 26.113) centre (62.2007, 8.0934) ccw projected
  arc A9 (25.7513, 47.9864) -> (20.7737, 44.9492) centre (28.245, 38.3023) ccw projected
  arc A10 (112.3783, 30.6103) -> (25.7513, 47.9864) centre (51.0785, -50.3709) ccw projected
  arc A11 (134.943, 0) -> (112.3783, 30.6103) centre (71.3369, -23.2658) ccw projected
  line L2 (144.468, 0) -> (134.943, 0) projected
  arc A12 (144.468, 0) -> (141.285, 9.525) centre (105.0517, -7.8776) ccw projected
  arc A13 (141.285, 9.525) -> (125.619, 31.7017) centre (71.3369, -23.2658) ccw projected
  line L3 (125.619, 31.7017) -> (125.619, 24.9245) projected
  line L4 (125.619, 24.9245) -> (122.571, 24.9245) projected
  line L5 (122.571, 24.9245) -> (122.571, 34.5532) projected
  arc A14 (122.571, 34.5532) -> (118.1386, 38.1962) centre (71.3369, -23.2658) ccw projected
  arc A15 (118.1386, 38.1962) -> (82.1543, 56.285) centre (51.0785, -50.3709) ccw projected
  line L6 (82.1543, 56.285) -> (82.1543, 50.421) projected
  line L7 (82.1543, 50.421) -> (79.1063, 50.421) projected
  line L8 (79.1063, 50.421) -> (79.1063, 57.1262) projected
  arc A16 (79.1063, 57.1262) -> (33.7295, 59.3569) centre (51.0785, -50.3709) ccw projected
  line L9 (33.7295, 59.3569) -> (33.7295, 52.94) projected
  line L10 (33.7295, 52.94) -> (30.6815, 52.94) projected
  point P0 (125.943, 0)
sketch "Sketch22" plane through (-2, 0, -92.2135) normal (0, 0, 1) x (1, 0, 0)
  line L0 (44.922, 52.94) -> (44.922, 59.3569) projected
  arc A0 (46.341, 52.1799) -> (44.922, 52.94) centre (42.3483, 46.4303) ccw projected
  arc A1 (69.05, 0) -> (46.341, 52.1799) centre (15.4585, 7.7082) ccw projected
  line L1 (78.575, 0) -> (69.05, 0) projected
  arc A2 (78.575, 0) -> (75.453, 28.8269) centre (-63.9548, -0.8536) ccw projected
  arc A3 (75.453, 28.8269) -> (75.1717, 29.7979) centre (68.6065, 27.3692) ccw projected
  arc A4 (75.1717, 29.7979) -> (51.774, 60.0035) centre (15.4585, 7.7082) ccw projected
  arc A5 (51.774, 60.0035) -> (48.0276, 61.9487) centre (42.3483, 46.4303) ccw projected
  arc A6 (48.0276, 61.9487) -> (29.65, 65.0829) centre (30.3196, 13.5622) ccw projected
  arc A7 (29.65, 65.0829) -> (11.2724, 61.9487) centre (28.9804, 13.5622) ccw projected
  arc A8 (11.2724, 61.9487) -> (7.526, 60.0035) centre (16.9517, 46.4303) ccw projected
  arc A9 (7.526, 60.0035) -> (-15.8717, 29.7979) centre (43.8415, 7.7082) ccw projected
  arc A10 (-15.8717, 29.7979) -> (-16.153, 28.8269) centre (-9.3065, 27.3692) ccw projected
  arc A11 (-16.153, 28.8269) -> (-19.275, 0) centre (123.2548, -0.8536) ccw projected
  line L2 (-9.75, 0) -> (-19.275, 0) projected
  arc A12 (12.959, 52.1799) -> (-9.75, 0) centre (43.8415, 7.7082) ccw projected
  arc A13 (14.378, 52.94) -> (12.959, 52.1799) centre (16.9517, 46.4303) ccw projected
  line L3 (14.378, 59.3569) -> (14.378, 52.94) projected
  line L4 (17.426, 59.3569) -> (14.378, 59.3569) projected
  line L5 (17.426, 53.9416) -> (17.426, 59.3569) projected
  arc A14 (29.65, 55.5569) -> (17.426, 53.9416) centre (28.9804, 13.5622) ccw projected
  arc A15 (41.874, 53.9416) -> (29.65, 55.5569) centre (30.3196, 13.5622) ccw projected
  line L6 (41.874, 59.3569) -> (41.874, 53.9416) projected
  line L7 (44.922, 59.3569) -> (41.874, 59.3569) projected
  point P0 (2, 0)
sketch "Sketch23" plane through (-2, 0, -43.7887) normal (0, 0, 1) x (1, 0, 0)
  line L0 (44.922, 50.4232) -> (44.922, 56.285) projected
  arc A0 (71.05, 0) -> (44.922, 50.4232) centre (30.5089, 10.9737) ccw projected
  line L1 (80.575, 0) -> (71.05, 0) projected
  arc A1 (80.575, 0) -> (74.4622, 37.8642) centre (9.7925, 7.9983) ccw projected
  arc A2 (74.4622, 37.8642) -> (28.0459, 62.4413) centre (30.5089, 10.9737) ccw projected
  arc A3 (28.0459, 62.4413) -> (-15.1613, 37.8649) centre (30.6726, 7.5545) ccw projected
  arc A4 (-15.1613, 37.8649) -> (-21.275, 0) centre (49.5076, 7.9974) ccw projected
  line L2 (-11.75, 0) -> (-21.275, 0) projected
  arc A5 (14.378, 50.421) -> (-11.75, 0) centre (28.7868, 10.9742) ccw projected
  line L3 (14.378, 56.285) -> (14.378, 50.421) projected
  line L4 (17.426, 56.285) -> (14.378, 56.285) projected
  line L5 (17.426, 51.4044) -> (17.426, 56.285) projected
  arc A6 (29.5626, 52.9631) -> (17.426, 51.4044) centre (28.7868, 10.9742) ccw projected
  arc A7 (41.874, 51.4068) -> (29.5626, 52.9631) centre (30.5089, 10.9737) ccw projected
  line L6 (41.874, 56.285) -> (41.874, 51.4068) projected
  line L7 (44.922, 56.285) -> (41.874, 56.285) projected
  point P0 (2, 0)
sketch "Sketch24" plane through (0, 0, -0.324) normal (0, 0, 1) x (1, 0, 0)
  line L0 (12.378, 31.7017) -> (12.378, 24.9245) projected
  line L1 (15.426, 31.7017) -> (12.378, 31.7017) projected
  line L2 (15.426, 26.2885) -> (15.426, 31.7017) projected
  arc A0 (29.345, 28.3859) -> (15.426, 26.2885) centre (27.0848, -3.85) ccw projected
  arc A1 (39.874, 26.2317) -> (29.345, 28.3859) centre (28.2224, -3.9096) ccw projected
  line L3 (39.874, 31.7017) -> (39.874, 26.2317) projected
  line L4 (42.922, 31.7017) -> (39.874, 31.7017) projected
  line L5 (42.922, 24.8685) -> (42.922, 31.7017) projected
  arc A2 (60.3, 0) -> (42.922, 24.8685) centre (28.2224, -3.9096) ccw projected
  line L6 (69.825, 0) -> (60.3, 0) projected
  arc A3 (69.825, 0) -> (67.8468, 9.525) centre (30.5982, -3.1788) ccw projected
  arc A4 (67.8468, 9.525) -> (29.6759, 37.9051) centre (28.2224, -3.9096) ccw projected
  arc A5 (29.6759, 37.9051) -> (25.6241, 37.9051) centre (27.65, 13.4592) ccw projected
  arc A6 (25.6241, 37.9051) -> (-12.5468, 9.525) centre (27.0776, -3.9096) ccw projected
  arc A7 (-12.5468, 9.525) -> (-14.525, 0) centre (24.7018, -3.1788) ccw projected
  line L7 (-5, 0) -> (-14.525, 0) projected
  arc A8 (12.378, 24.9245) -> (-5, 0) centre (27.0848, -3.85) ccw projected
  point P0 (0, 0)
body "Solid1"
